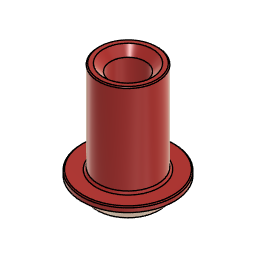
Capuchon_Prise_Jack_Onduleur (Autodesk Fusion 360 design; units mm, degrees)
Autodesk Fusion 360 part; units mm, degrees
sketch "Esquisse1" plane through (0, 0, 0) normal (0, 0, 1) x (1, 0, 0)
  circle A0 centre (0, 0) radius 4.5
  circle A1 centre (0, 0) radius 2.9
  circle A2 centre (0, 0) radius 1.7
  dimension "d1" = 5.8
  dimension "d2" = 3.4
  dimension "d3" = 9
  constraint coincident A0.centre A1.centre
  constraint concentric A1 A2
  measures "d1" diameter of A1
  measures "d2" diameter of A2
  measures "d3" diameter of A0
extrude "Extrusion1" add sketch "Esquisse1" along normal blind 9 contours A1
extrude "Extrusion2" add sketch "Esquisse1" against normal blind 2 contours A0 | A1 | A2
chamfer "Chanfrein1" distance 1 angle 45 1 edges at (-1.585, 0.6147, 0)
chamfer "Chanfrein2" distance 1.5 angle 45 1 edges at (-4.1955, 1.6273, -2)
chamfer "Chanfrein3" distance 0.7 angle 45 1 edges at (-1.585, 0.6147, 9)
chamfer "Chanfrein4" distance 0.1 angle 45 1 edges at (-2.7037, -1.0487, 9)
chamfer "Chanfrein5" distance 0.1 angle 45 1 edges at (-4.1955, -1.6273, 0)
chamfer "Chanfrein6" distance 0.2 angle 45 1 edges at (-2.7037, -1.0487, 0)
